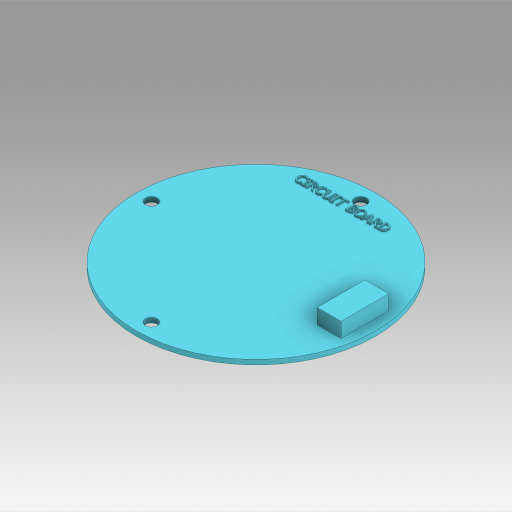
# Autodesk Inventor part: ROUNDPCB
Saved by Autodesk Inventor 2023 (Build 270158000, 158)
## iProperties
Created: 2025-09-17
Part Number: ROUNDPCB
Material: Generic
Document SubType Name: Modeling
Designer: NELLY NDUNG'U
Density: 1 g/cm^3
Appearance: Cadet Blue
Author: NELLY NDUNG'U
Autodesk Inventor part; units mm, degrees
ref_plane "YZ Plane" through (0, 0, 0) normal (1, 0, 0) x (0, 1, 0)
ref_plane "XZ Plane" through (0, 0, 0) normal (0, 1, 0) x (-1, 0, 0)
ref_plane "XY Plane" through (0, 0, 0) normal (0, 0, 1) x (1, 0, 0)
sketch "Sketch1" plane through (0, 0, 0) normal (0, 1, 0) x (-1, 0, 0)
  circle A0 centre (0, 0) radius 40
  dimension "d0" = 80
  constraints: 1 centre point, 1 coincident
  measures "d0" diameter of A0
extrude "Extrusion1" add sketch "Sketch1" along normal blind 1.6
sketch "Sketch2" plane through (0, 1.6, 0) normal (0, 1, 0) x (1, 0, 0)
  line L0 (28.45, -8) -> (36.45, -8)
  line L1 (36.45, -8) -> (36.45, 8)
  line L2 (36.45, 8) -> (28.45, 8)
  line L3 (28.45, 8) -> (28.45, -8)
  circle A0 centre (0, 0) radius 40 projected
  line L4 (0, 0) -> (40, 0) construction
  circle A1 centre (0, 0) radius 40 projected
  point P0 (36.45, 0)
  dimension "d3" = 16
  dimension "d4" = 36.45
  dimension "d5" = 8
  constraints: 10 end point, 2 horizontal, 2 parallel, 1 horizontal alignment, 1 midpoint, 1 perpendicular, 2 other
  measures "d3" distance of L2.end L0.start
  measures "d4" distance of L4.start point (36.45, 0)
  measures "d5" distance of L0.start L0.end
extrude "Extrusion2" add sketch "Sketch2" along normal blind 5 contours L3 L2 L1 L0
sketch "Sketch3" plane through (0, 1.6, 0) normal (0, 1, 0) x (1, 0, 0)
  line L0 (-17.4643, 32.8011) -> (13.1985, 32.8011) construction
  line L1 (13.1985, 32.8011) -> (13.1985, 29.6247) construction
  line L2 (13.1985, 29.6247) -> (-17.4643, 29.6247) construction
  line L3 (-17.4643, 29.6247) -> (-17.4643, 32.8011) construction
  circle A0 centre (0, 0) radius 40 construction
  spline S0 degree 2 poles (-15.965, 29.6345) (-16.2614, 29.6345) (-16.7628, 29.8346) (-16.9456, 30.0347) knots 0 0 0 1 2 2 2
  spline S1 degree 2 poles (-16.9456, 30.0347) (-17.1283, 30.2323) (-17.3284, 30.8251) (-17.3284, 31.2104) knots 0 0 0 1 2 2 2
  spline S2 degree 2 poles (-17.3284, 31.2104) (-17.3284, 31.5933) (-17.1333, 32.1614) (-16.948, 32.3713) knots 0 0 0 1 2 2 2
  spline S3 degree 2 poles (-16.948, 32.3713) (-16.7653, 32.5763) (-16.2663, 32.7912) (-15.9576, 32.7912) knots 0 0 0 1 2 2 2
  spline S4 degree 2 poles (-15.9576, 32.7912) (-15.8044, 32.7912) (-15.5352, 32.7468) (-15.4216, 32.7122) knots 0 0 0 1 2 2 2
  spline S5 degree 2 poles (-15.4216, 32.7122) (-15.3228, 32.6801) (-15.1178, 32.5887) (-15.0165, 32.5343) knots 0 0 0 1 2 2 2
  line L4 (-15.0165, 32.5343) -> (-15.0165, 32.0453)
  line L5 (-15.0165, 32.0453) -> (-15.0486, 32.0453)
  spline S6 degree 2 poles (-15.0486, 32.0453) (-15.1029, 32.0947) (-15.2709, 32.233) (-15.3919, 32.2997) knots 0 0 0 1 2 2 2
  spline S7 degree 2 poles (-15.3919, 32.2997) (-15.508, 32.3639) (-15.7822, 32.4454) (-15.96, 32.4454) knots 0 0 0 1 2 2 2
  spline S8 degree 2 poles (-15.96, 32.4454) (-16.1552, 32.4454) (-16.5034, 32.2849) (-16.6343, 32.1317) knots 0 0 0 1 2 2 2
  spline S9 degree 2 poles (-16.6343, 32.1317) (-16.7628, 31.9761) (-16.906, 31.5044) (-16.906, 31.2104) knots 0 0 0 1 2 2 2
  spline S10 degree 2 poles (-16.906, 31.2104) (-16.906, 30.8967) (-16.7554, 30.4447) (-16.6245, 30.2891) knots 0 0 0 1 2 2 2
  spline S11 degree 2 poles (-16.6245, 30.2891) (-16.496, 30.1384) (-16.1527, 29.9853) (-15.96, 29.9853) knots 0 0 0 1 2 2 2
  spline S12 degree 2 poles (-15.96, 29.9853) (-15.7847, 29.9853) (-15.4858, 30.0717) (-15.3697, 30.136) knots 0 0 0 1 2 2 2
  spline S13 degree 2 poles (-15.3697, 30.136) (-15.2585, 30.2002) (-15.0931, 30.3336) (-15.0461, 30.3805) knots 0 0 0 1 2 2 2
  line L6 (-15.0461, 30.3805) -> (-15.0165, 30.3805)
  line L7 (-15.0165, 30.3805) -> (-15.0165, 29.8964)
  spline S14 degree 2 poles (-15.0165, 29.8964) (-15.1178, 29.8494) (-15.2956, 29.763) (-15.4216, 29.7235) knots 0 0 0 1 2 2 2
  spline S15 degree 2 poles (-15.4216, 29.7235) (-15.5549, 29.679) (-15.7822, 29.6345) (-15.965, 29.6345) knots 0 0 0 1 2 2 2
  line L8 (-13.5765, 29.6889) -> (-14.7571, 29.6889)
  line L9 (-14.7571, 29.6889) -> (-14.7571, 30.0001)
  line L10 (-14.7571, 30.0001) -> (-14.3693, 30.0001)
  line L11 (-14.3693, 30.0001) -> (-14.3693, 32.4257)
  line L12 (-14.3693, 32.4257) -> (-14.7571, 32.4257)
  line L13 (-14.7571, 32.4257) -> (-14.7571, 32.7369)
  line L14 (-14.7571, 32.7369) -> (-13.5765, 32.7369)
  line L15 (-13.5765, 32.7369) -> (-13.5765, 32.4257)
  line L16 (-13.5765, 32.4257) -> (-13.9643, 32.4257)
  line L17 (-13.9643, 32.4257) -> (-13.9643, 30.0001)
  line L18 (-13.9643, 30.0001) -> (-13.5765, 30.0001)
  line L19 (-13.5765, 30.0001) -> (-13.5765, 29.6889)
  line L20 (-10.7162, 29.6889) -> (-11.2423, 29.6889)
  line L21 (-11.2423, 29.6889) -> (-12.2056, 30.9017)
  line L22 (-12.2056, 30.9017) -> (-12.67, 30.9017)
  line L23 (-12.67, 30.9017) -> (-12.67, 29.6889)
  line L24 (-12.67, 29.6889) -> (-13.0751, 29.6889)
  line L25 (-13.0751, 29.6889) -> (-13.0751, 32.7369)
  line L26 (-13.0751, 32.7369) -> (-12.2896, 32.7369)
  spline S16 degree 2 poles (-12.2896, 32.7369) (-12.0278, 32.7369) (-11.6746, 32.6801) (-11.514, 32.5763) knots 0 0 0 1 2 2 2
  spline S17 degree 2 poles (-11.514, 32.5763) (-11.3535, 32.4726) (-11.1682, 32.149) (-11.1682, 31.9094) knots 0 0 0 1 2 2 2
  spline S18 degree 2 poles (-11.1682, 31.9094) (-11.1682, 31.576) (-11.5091, 31.124) (-11.8005, 31.0153) knots 0 0 0 1 2 2 2
  line L27 (-11.8005, 31.0153) -> (-10.7162, 29.6889)
  spline S19 degree 2 poles (-11.5906, 31.8773) (-11.5906, 32.0107) (-11.6844, 32.2157) (-11.7832, 32.2824) knots 0 0 0 1 2 2 2
  spline S20 degree 2 poles (-11.7832, 32.2824) (-11.8697, 32.3392) (-12.0994, 32.3861) (-12.2674, 32.3861) knots 0 0 0 1 2 2 2
  line L28 (-12.2674, 32.3861) -> (-12.67, 32.3861)
  line L29 (-12.67, 32.3861) -> (-12.67, 31.2401)
  line L30 (-12.67, 31.2401) -> (-12.3143, 31.2401)
  spline S21 degree 2 poles (-12.3143, 31.2401) (-12.1389, 31.2401) (-11.8598, 31.3018) (-11.7635, 31.3981) knots 0 0 0 1 2 2 2
  spline S22 degree 2 poles (-11.7635, 31.3981) (-11.6746, 31.4821) (-11.5906, 31.7192) (-11.5906, 31.8773) knots 0 0 0 1 2 2 2
  spline S23 degree 2 poles (-9.2836, 29.6345) (-9.58, 29.6345) (-10.0814, 29.8346) (-10.2642, 30.0347) knots 0 0 0 1 2 2 2
  spline S24 degree 2 poles (-10.2642, 30.0347) (-10.447, 30.2323) (-10.647, 30.8251) (-10.647, 31.2104) knots 0 0 0 1 2 2 2
  spline S25 degree 2 poles (-10.647, 31.2104) (-10.647, 31.5933) (-10.4519, 32.1614) (-10.2666, 32.3713) knots 0 0 0 1 2 2 2
  spline S26 degree 2 poles (-10.2666, 32.3713) (-10.0839, 32.5763) (-9.5849, 32.7912) (-9.2762, 32.7912) knots 0 0 0 1 2 2 2
  spline S27 degree 2 poles (-9.2762, 32.7912) (-9.123, 32.7912) (-8.8538, 32.7468) (-8.7402, 32.7122) knots 0 0 0 1 2 2 2
  spline S28 degree 2 poles (-8.7402, 32.7122) (-8.6414, 32.6801) (-8.4364, 32.5887) (-8.3351, 32.5343) knots 0 0 0 1 2 2 2
  line L31 (-8.3351, 32.5343) -> (-8.3351, 32.0453)
  line L32 (-8.3351, 32.0453) -> (-8.3672, 32.0453)
  spline S29 degree 2 poles (-8.3672, 32.0453) (-8.4215, 32.0947) (-8.5895, 32.233) (-8.7105, 32.2997) knots 0 0 0 1 2 2 2
  spline S30 degree 2 poles (-8.7105, 32.2997) (-8.8266, 32.3639) (-9.1008, 32.4454) (-9.2786, 32.4454) knots 0 0 0 1 2 2 2
  spline S31 degree 2 poles (-9.2786, 32.4454) (-9.4738, 32.4454) (-9.822, 32.2849) (-9.953, 32.1317) knots 0 0 0 1 2 2 2
  spline S32 degree 2 poles (-9.953, 32.1317) (-10.0814, 31.9761) (-10.2247, 31.5044) (-10.2247, 31.2104) knots 0 0 0 1 2 2 2
  spline S33 degree 2 poles (-10.2247, 31.2104) (-10.2247, 30.8967) (-10.074, 30.4447) (-9.9431, 30.2891) knots 0 0 0 1 2 2 2
  spline S34 degree 2 poles (-9.9431, 30.2891) (-9.8146, 30.1384) (-9.4713, 29.9853) (-9.2786, 29.9853) knots 0 0 0 1 2 2 2
  spline S35 degree 2 poles (-9.2786, 29.9853) (-9.1033, 29.9853) (-8.8044, 30.0717) (-8.6883, 30.136) knots 0 0 0 1 2 2 2
  spline S36 degree 2 poles (-8.6883, 30.136) (-8.5772, 30.2002) (-8.4117, 30.3336) (-8.3647, 30.3805) knots 0 0 0 1 2 2 2
  line L33 (-8.3647, 30.3805) -> (-8.3351, 30.3805)
  line L34 (-8.3351, 30.3805) -> (-8.3351, 29.8964)
  spline S37 degree 2 poles (-8.3351, 29.8964) (-8.4364, 29.8494) (-8.6142, 29.763) (-8.7402, 29.7235) knots 0 0 0 1 2 2 2
  spline S38 degree 2 poles (-8.7402, 29.7235) (-8.8736, 29.679) (-9.1008, 29.6345) (-9.2836, 29.6345) knots 0 0 0 1 2 2 2
  spline S39 degree 2 poles (-6.8926, 29.6247) (-7.1618, 29.6247) (-7.562, 29.7655) (-7.7028, 29.9063) knots 0 0 0 1 2 2 2
  spline S40 degree 2 poles (-7.7028, 29.9063) (-7.8633, 30.0643) (-7.9942, 30.5089) (-7.9942, 30.835) knots 0 0 0 1 2 2 2
  line L35 (-7.9942, 30.835) -> (-7.9942, 32.7369)
  line L36 (-7.9942, 32.7369) -> (-7.5891, 32.7369)
  line L37 (-7.5891, 32.7369) -> (-7.5891, 30.835)
  spline S41 degree 2 poles (-7.5891, 30.835) (-7.5891, 30.6226) (-7.5348, 30.336) (-7.4582, 30.2199) knots 0 0 0 1 2 2 2
  spline S42 degree 2 poles (-7.4582, 30.2199) (-7.3767, 30.0964) (-7.0951, 29.9705) (-6.8926, 29.9705) knots 0 0 0 1 2 2 2
  spline S43 degree 2 poles (-6.8926, 29.9705) (-6.7024, 29.9705) (-6.406, 30.0964) (-6.3245, 30.2199) knots 0 0 0 1 2 2 2
  spline S44 degree 2 poles (-6.3245, 30.2199) (-6.2479, 30.336) (-6.1936, 30.6201) (-6.1936, 30.8251) knots 0 0 0 1 2 2 2
  line L38 (-6.1936, 30.8251) -> (-6.1936, 32.7369)
  line L39 (-6.1936, 32.7369) -> (-5.7885, 32.7369)
  line L40 (-5.7885, 32.7369) -> (-5.7885, 30.835)
  spline S45 degree 2 poles (-5.7885, 30.835) (-5.7885, 30.5163) (-5.9169, 30.0619) (-6.08, 29.9063) knots 0 0 0 1 2 2 2
  spline S46 degree 2 poles (-6.08, 29.9063) (-6.2257, 29.763) (-6.611, 29.6247) (-6.8926, 29.6247) knots 0 0 0 1 2 2 2
  line L41 (-4.1459, 29.6889) -> (-5.3266, 29.6889)
  line L42 (-5.3266, 29.6889) -> (-5.3266, 30.0001)
  line L43 (-5.3266, 30.0001) -> (-4.9388, 30.0001)
  line L44 (-4.9388, 30.0001) -> (-4.9388, 32.4257)
  line L45 (-4.9388, 32.4257) -> (-5.3266, 32.4257)
  line L46 (-5.3266, 32.4257) -> (-5.3266, 32.7369)
  line L47 (-5.3266, 32.7369) -> (-4.1459, 32.7369)
  line L48 (-4.1459, 32.7369) -> (-4.1459, 32.4257)
  line L49 (-4.1459, 32.4257) -> (-4.5337, 32.4257)
  line L50 (-4.5337, 32.4257) -> (-4.5337, 30.0001)
  line L51 (-4.5337, 30.0001) -> (-4.1459, 30.0001)
  line L52 (-4.1459, 30.0001) -> (-4.1459, 29.6889)
  line L53 (-2.9332, 29.6889) -> (-2.9332, 32.3763)
  line L54 (-2.9332, 32.3763) -> (-3.9558, 32.3763)
  line L55 (-3.9558, 32.3763) -> (-3.9558, 32.7369)
  line L56 (-3.9558, 32.7369) -> (-1.5055, 32.7369)
  line L57 (-1.5055, 32.7369) -> (-1.5055, 32.3763)
  line L58 (-1.5055, 32.3763) -> (-2.5281, 32.3763)
  line L59 (-2.5281, 32.3763) -> (-2.5281, 29.6889)
  line L60 (-2.5281, 29.6889) -> (-2.9332, 29.6889)
  spline S47 degree 2 poles (2.1798, 30.625) (2.1798, 30.3978) (2.0069, 30.0495) (1.8636, 29.9359) knots 0 0 0 1 2 2 2
  spline S48 degree 2 poles (1.8636, 29.9359) (1.6907, 29.8025) (1.298, 29.6889) (0.9867, 29.6889) knots 0 0 0 1 2 2 2
  line L61 (0.9867, 29.6889) -> (0.1124, 29.6889)
  line L62 (0.1124, 29.6889) -> (0.1124, 32.7369)
  line L63 (0.1124, 32.7369) -> (0.9201, 32.7369)
  spline S49 degree 2 poles (0.9201, 32.7369) (1.2461, 32.7369) (1.5721, 32.6949) (1.7203, 32.6134) knots 0 0 0 1 2 2 2
  spline S50 degree 2 poles (1.7203, 32.6134) (1.8858, 32.5269) (2.0365, 32.2429) (2.0365, 32.0502) knots 0 0 0 1 2 2 2
  spline S51 degree 2 poles (2.0365, 32.0502) (2.0365, 31.8353) (1.8093, 31.4945) (1.6092, 31.3981) knots 0 0 0 1 2 2 2
  line L64 (1.6092, 31.3981) -> (1.6092, 31.3833)
  spline S52 degree 2 poles (1.6092, 31.3833) (1.8809, 31.3092) (2.1798, 30.9165) (2.1798, 30.625) knots 0 0 0 1 2 2 2
  spline S53 degree 2 poles (1.7574, 30.6077) (1.7574, 30.7806) (1.6586, 31.0029) (1.5104, 31.082) knots 0 0 0 1 2 2 2
  spline S54 degree 2 poles (1.5104, 31.082) (1.4141, 31.1314) (1.1868, 31.161) (0.9769, 31.161) knots 0 0 0 1 2 2 2
  line L65 (0.9769, 31.161) -> (0.5174, 31.161)
  line L66 (0.5174, 31.161) -> (0.5174, 30.0347)
  line L67 (0.5174, 30.0347) -> (0.846, 30.0347)
  spline S55 degree 2 poles (0.846, 30.0347) (1.1127, 30.0347) (1.419, 30.0841) (1.5376, 30.1631) knots 0 0 0 1 2 2 2
  spline S56 degree 2 poles (1.5376, 30.1631) (1.6512, 30.2446) (1.7574, 30.4472) (1.7574, 30.6077) knots 0 0 0 1 2 2 2
  spline S57 degree 2 poles (1.6141, 31.9934) (1.6141, 32.1021) (1.54, 32.2651) (1.4585, 32.312) knots 0 0 0 1 2 2 2
  spline S58 degree 2 poles (1.4585, 32.312) (1.3597, 32.3664) (1.1201, 32.3911) (0.9052, 32.3911) knots 0 0 0 1 2 2 2
  line L68 (0.9052, 32.3911) -> (0.5174, 32.3911)
  line L69 (0.5174, 32.3911) -> (0.5174, 31.4994)
  line L70 (0.5174, 31.4994) -> (0.9769, 31.4994)
  spline S59 degree 2 poles (0.9769, 31.4994) (1.1671, 31.4994) (1.3474, 31.5389) (1.4437, 31.6007) knots 0 0 0 1 2 2 2
  spline S60 degree 2 poles (1.4437, 31.6007) (1.5376, 31.66) (1.6141, 31.8502) (1.6141, 31.9934) knots 0 0 0 1 2 2 2
  spline S61 degree 2 poles (4.7387, 32.3886) (4.9116, 32.1861) (5.1043, 31.5933) (5.1043, 31.2129) knots 0 0 0 1 2 2 2
  spline S62 degree 2 poles (5.1043, 31.2129) (5.1043, 30.8424) (4.9165, 30.2422) (4.7387, 30.0396) knots 0 0 0 1 2 2 2
  spline S63 degree 2 poles (4.7387, 30.0396) (4.551, 29.8272) (4.0545, 29.6247) (3.7556, 29.6247) knots 0 0 0 1 2 2 2
  spline S64 degree 2 poles (3.7556, 29.6247) (3.4469, 29.6247) (2.9529, 29.8346) (2.7726, 30.0396) knots 0 0 0 1 2 2 2
  spline S65 degree 2 poles (2.7726, 30.0396) (2.5972, 30.2422) (2.4095, 30.8374) (2.4095, 31.2129) knots 0 0 0 1 2 2 2
  spline S66 degree 2 poles (2.4095, 31.2129) (2.4095, 31.5957) (2.5997, 32.1787) (2.775, 32.3886) knots 0 0 0 1 2 2 2
  spline S67 degree 2 poles (2.775, 32.3886) (2.9529, 32.5912) (3.4494, 32.8011) (3.7556, 32.8011) knots 0 0 0 1 2 2 2
  spline S68 degree 2 poles (3.7556, 32.8011) (4.0669, 32.8011) (4.5658, 32.5837) (4.7387, 32.3886) knots 0 0 0 1 2 2 2
  spline S69 degree 2 poles (4.6819, 31.2129) (4.6819, 31.5142) (4.551, 31.9811) (4.4324, 32.1342) knots 0 0 0 1 2 2 2
  spline S70 degree 2 poles (4.4324, 32.1342) (4.3114, 32.2923) (3.9705, 32.4504) (3.7581, 32.4504) knots 0 0 0 1 2 2 2
  spline S71 degree 2 poles (3.7581, 32.4504) (3.5383, 32.4504) (3.2073, 32.2972) (3.0813, 32.1342) knots 0 0 0 1 2 2 2
  spline S72 degree 2 poles (3.0813, 32.1342) (2.9603, 31.9786) (2.8319, 31.5093) (2.8319, 31.2129) knots 0 0 0 1 2 2 2
  spline S73 degree 2 poles (2.8319, 31.2129) (2.8319, 30.6127) (3.3357, 29.9754) (3.7581, 29.9754) knots 0 0 0 1 2 2 2
  spline S74 degree 2 poles (3.7581, 29.9754) (4.1805, 29.9754) (4.6819, 30.6127) (4.6819, 31.2129) knots 0 0 0 1 2 2 2
  line L71 (5.2204, 29.6889) -> (6.2479, 32.7369)
  line L72 (6.2479, 32.7369) -> (6.7468, 32.7369)
  line L73 (6.7468, 32.7369) -> (7.7744, 29.6889)
  line L74 (7.7744, 29.6889) -> (7.347, 29.6889)
  line L75 (7.347, 29.6889) -> (7.0704, 30.541)
  line L76 (7.0704, 30.541) -> (5.907, 30.541)
  line L77 (5.907, 30.541) -> (5.6304, 29.6889)
  line L78 (5.6304, 29.6889) -> (5.2204, 29.6889)
  line L79 (6.9592, 30.8868) -> (6.4875, 32.3219)
  line L80 (6.4875, 32.3219) -> (6.0182, 30.8868)
  line L81 (6.0182, 30.8868) -> (6.9592, 30.8868)
  line L82 (10.4222, 29.6889) -> (9.8961, 29.6889)
  line L83 (9.8961, 29.6889) -> (8.9328, 30.9017)
  line L84 (8.9328, 30.9017) -> (8.4684, 30.9017)
  line L85 (8.4684, 30.9017) -> (8.4684, 29.6889)
  line L86 (8.4684, 29.6889) -> (8.0633, 29.6889)
  line L87 (8.0633, 29.6889) -> (8.0633, 32.7369)
  line L88 (8.0633, 32.7369) -> (8.8488, 32.7369)
  spline S75 degree 2 poles (8.8488, 32.7369) (9.1106, 32.7369) (9.4638, 32.6801) (9.6244, 32.5763) knots 0 0 0 1 2 2 2
  spline S76 degree 2 poles (9.6244, 32.5763) (9.7849, 32.4726) (9.9702, 32.149) (9.9702, 31.9094) knots 0 0 0 1 2 2 2
  spline S77 degree 2 poles (9.9702, 31.9094) (9.9702, 31.576) (9.6293, 31.124) (9.3379, 31.0153) knots 0 0 0 1 2 2 2
  line L89 (9.3379, 31.0153) -> (10.4222, 29.6889)
  spline S78 degree 2 poles (9.5478, 31.8773) (9.5478, 32.0107) (9.454, 32.2157) (9.3552, 32.2824) knots 0 0 0 1 2 2 2
  spline S79 degree 2 poles (9.3552, 32.2824) (9.2687, 32.3392) (9.039, 32.3861) (8.871, 32.3861) knots 0 0 0 1 2 2 2
  line L90 (8.871, 32.3861) -> (8.4684, 32.3861)
  line L91 (8.4684, 32.3861) -> (8.4684, 31.2401)
  line L92 (8.4684, 31.2401) -> (8.8241, 31.2401)
  spline S80 degree 2 poles (8.8241, 31.2401) (8.9995, 31.2401) (9.2786, 31.3018) (9.3749, 31.3981) knots 0 0 0 1 2 2 2
  spline S81 degree 2 poles (9.3749, 31.3981) (9.4638, 31.4821) (9.5478, 31.7192) (9.5478, 31.8773) knots 0 0 0 1 2 2 2
  spline S82 degree 2 poles (13.0676, 31.2104) (13.0676, 30.793) (12.7292, 30.1211) (12.4452, 29.9334) knots 0 0 0 1 2 2 2
  spline S83 degree 2 poles (12.4452, 29.9334) (12.213, 29.7877) (11.7363, 29.6889) (11.3658, 29.6889) knots 0 0 0 1 2 2 2
  line L93 (11.3658, 29.6889) -> (10.6643, 29.6889)
  line L94 (10.6643, 29.6889) -> (10.6643, 32.7369)
  line L95 (10.6643, 32.7369) -> (11.3583, 32.7369)
  spline S84 degree 2 poles (11.3583, 32.7369) (11.7881, 32.7369) (12.2772, 32.6084) (12.4501, 32.4948) knots 0 0 0 1 2 2 2
  spline S85 degree 2 poles (12.4501, 32.4948) (12.744, 32.2997) (13.0676, 31.655) (13.0676, 31.2104) knots 0 0 0 1 2 2 2
  spline S86 degree 2 poles (12.6452, 31.2154) (12.6452, 31.5661) (12.413, 32.0626) (12.1833, 32.2034) knots 0 0 0 1 2 2 2
  spline S87 degree 2 poles (12.1833, 32.2034) (12.0203, 32.2997) (11.6523, 32.3861) (11.3781, 32.3861) knots 0 0 0 1 2 2 2
  line L96 (11.3781, 32.3861) -> (11.0694, 32.3861)
  line L97 (11.0694, 32.3861) -> (11.0694, 30.0396)
  line L98 (11.0694, 30.0396) -> (11.3781, 30.0396)
  spline S88 degree 2 poles (11.3781, 30.0396) (11.6473, 30.0396) (12.0549, 30.1261) (12.2204, 30.2422) knots 0 0 0 1 2 2 2
  spline S89 degree 2 poles (12.2204, 30.2422) (12.4328, 30.3854) (12.6452, 30.8597) (12.6452, 31.2154) knots 0 0 0 1 2 2 2
  constraints: 2 other
emboss "Emboss1" sketch "Sketch3" operation add depth 0.5 direction (0, -1, 0)
sketch "Sketch4" plane through (0, 1.6, 0) normal (0, 1, 0) x (1, 0, 0)
  circle A0 centre (0, 0) radius 40 projected
  line L0 (36.45, -8) -> (28.45, -8) projected
  line L1 (28.45, -8) -> (28.45, 8) projected
  line L2 (28.45, 8) -> (36.45, 8) projected
  line L3 (36.45, 8) -> (36.45, -8) projected
  line L4 (10.6643, 32.7369) -> (11.3583, 32.7369) projected
  line L5 (11.3658, 29.6889) -> (10.6643, 29.6889) projected
  line L6 (10.6643, 29.6889) -> (10.6643, 32.7369) projected
  line L7 (-4.1459, 32.4257) -> (-4.5337, 32.4257) projected
  line L8 (-4.5337, 32.4257) -> (-4.5337, 30.0001) projected
  line L9 (-4.5337, 30.0001) -> (-4.1459, 30.0001) projected
  line L10 (-4.1459, 30.0001) -> (-4.1459, 29.6889) projected
  line L11 (-4.1459, 29.6889) -> (-5.3266, 29.6889) projected
  line L12 (-5.3266, 29.6889) -> (-5.3266, 30.0001) projected
  line L13 (-5.3266, 30.0001) -> (-4.9388, 30.0001) projected
  line L14 (-4.9388, 30.0001) -> (-4.9388, 32.4257) projected
  line L15 (-4.9388, 32.4257) -> (-5.3266, 32.4257) projected
  line L16 (-5.3266, 32.4257) -> (-5.3266, 32.7369) projected
  line L17 (-5.3266, 32.7369) -> (-4.1459, 32.7369) projected
  line L18 (-4.1459, 32.7369) -> (-4.1459, 32.4257) projected
  line L19 (8.0633, 32.7369) -> (8.8488, 32.7369) projected
  line L20 (9.3379, 31.0153) -> (10.4222, 29.6889) projected
  line L21 (10.4222, 29.6889) -> (9.8961, 29.6889) projected
  line L22 (9.8961, 29.6889) -> (8.9328, 30.9017) projected
  line L23 (8.9328, 30.9017) -> (8.4684, 30.9017) projected
  line L24 (8.4684, 30.9017) -> (8.4684, 29.6889) projected
  line L25 (8.4684, 29.6889) -> (8.0633, 29.6889) projected
  line L26 (8.0633, 29.6889) -> (8.0633, 32.7369) projected
  line L27 (-8.3647, 30.3805) -> (-8.3351, 30.3805) projected
  line L28 (-8.3351, 30.3805) -> (-8.3351, 29.8964) projected
  line L29 (-8.3351, 32.5343) -> (-8.3351, 32.0453) projected
  line L30 (-8.3351, 32.0453) -> (-8.3672, 32.0453) projected
  line L31 (7.0704, 30.541) -> (5.907, 30.541) projected
  line L32 (5.907, 30.541) -> (5.6304, 29.6889) projected
  line L33 (5.6304, 29.6889) -> (5.2204, 29.6889) projected
  line L34 (5.2204, 29.6889) -> (6.2479, 32.7369) projected
  line L35 (6.2479, 32.7369) -> (6.7468, 32.7369) projected
  line L36 (6.7468, 32.7369) -> (7.7744, 29.6889) projected
  line L37 (7.7744, 29.6889) -> (7.347, 29.6889) projected
  line L38 (7.347, 29.6889) -> (7.0704, 30.541) projected
  line L39 (-11.8005, 31.0153) -> (-10.7162, 29.6889) projected
  line L40 (-10.7162, 29.6889) -> (-11.2423, 29.6889) projected
  line L41 (-11.2423, 29.6889) -> (-12.2056, 30.9017) projected
  line L42 (-12.2056, 30.9017) -> (-12.67, 30.9017) projected
  line L43 (-12.67, 30.9017) -> (-12.67, 29.6889) projected
  line L44 (-12.67, 29.6889) -> (-13.0751, 29.6889) projected
  line L45 (-13.0751, 29.6889) -> (-13.0751, 32.7369) projected
  line L46 (-13.0751, 32.7369) -> (-12.2896, 32.7369) projected
  line L47 (-15.0461, 30.3805) -> (-15.0165, 30.3805) projected
  line L48 (-15.0165, 30.3805) -> (-15.0165, 29.8964) projected
  line L49 (-15.0165, 32.5343) -> (-15.0165, 32.0453) projected
  line L50 (-15.0165, 32.0453) -> (-15.0486, 32.0453) projected
  line L51 (-1.5055, 32.3763) -> (-2.5281, 32.3763) projected
  line L52 (-2.5281, 32.3763) -> (-2.5281, 29.6889) projected
  line L53 (-2.5281, 29.6889) -> (-2.9332, 29.6889) projected
  line L54 (-2.9332, 29.6889) -> (-2.9332, 32.3763) projected
  line L55 (-2.9332, 32.3763) -> (-3.9558, 32.3763) projected
  line L56 (-3.9558, 32.3763) -> (-3.9558, 32.7369) projected
  line L57 (-3.9558, 32.7369) -> (-1.5055, 32.7369) projected
  line L58 (-1.5055, 32.7369) -> (-1.5055, 32.3763) projected
  line L59 (-13.5765, 32.4257) -> (-13.9643, 32.4257) projected
  line L60 (-13.9643, 32.4257) -> (-13.9643, 30.0001) projected
  line L61 (-13.9643, 30.0001) -> (-13.5765, 30.0001) projected
  line L62 (-13.5765, 30.0001) -> (-13.5765, 29.6889) projected
  line L63 (-13.5765, 29.6889) -> (-14.7571, 29.6889) projected
  line L64 (-14.7571, 29.6889) -> (-14.7571, 30.0001) projected
  line L65 (-14.7571, 30.0001) -> (-14.3693, 30.0001) projected
  line L66 (-14.3693, 30.0001) -> (-14.3693, 32.4257) projected
  line L67 (-14.3693, 32.4257) -> (-14.7571, 32.4257) projected
  line L68 (-14.7571, 32.4257) -> (-14.7571, 32.7369) projected
  line L69 (-14.7571, 32.7369) -> (-13.5765, 32.7369) projected
  line L70 (-13.5765, 32.7369) -> (-13.5765, 32.4257) projected
  line L71 (-6.1936, 30.8251) -> (-6.1936, 32.7369) projected
  line L72 (-6.1936, 32.7369) -> (-5.7885, 32.7369) projected
  line L73 (-5.7885, 32.7369) -> (-5.7885, 30.835) projected
  line L74 (-7.9942, 30.835) -> (-7.9942, 32.7369) projected
  line L75 (-7.9942, 32.7369) -> (-7.5891, 32.7369) projected
  line L76 (-7.5891, 32.7369) -> (-7.5891, 30.835) projected
  line L77 (1.6092, 31.3981) -> (1.6092, 31.3833) projected
  line L78 (0.9867, 29.6889) -> (0.1124, 29.6889) projected
  line L79 (0.1124, 29.6889) -> (0.1124, 32.7369) projected
  line L80 (0.1124, 32.7369) -> (0.9201, 32.7369) projected
  circle A1 centre (0, 0) radius 40 projected
  line L81 (0, -40) -> (0, 0) construction
  line L82 (0, 0) -> (-40, 0) construction
  circle A2 centre (0, -35) radius 2
  circle A3 centre (-35, 0) radius 2
  line L83 (0, 0) -> (0, 40) construction
  circle A4 centre (0, 35) radius 2
  dimension "d16" = 4
  dimension "d17" = 5
  dimension "d18" = 4
  dimension "d19" = 5
  dimension "d20" = 4
  dimension "d21" = 5
  constraints: 6 end point, 3 centre point, 3 point on circle, 3 point on line, 2 vertical, 1 perpendicular, 64 other
  measures "d16" diameter of A2
  measures "d17" distance of A2.centre L81.start
  measures "d18" diameter of A3
  measures "d19" distance of L82.end A3.centre
  measures "d20" diameter of A4
  measures "d21" distance of L83.end A4.centre
extrude "Extrusion3" cut sketch "Sketch4" against normal through all contours A2 | A3 | A4
body "Solid1"
